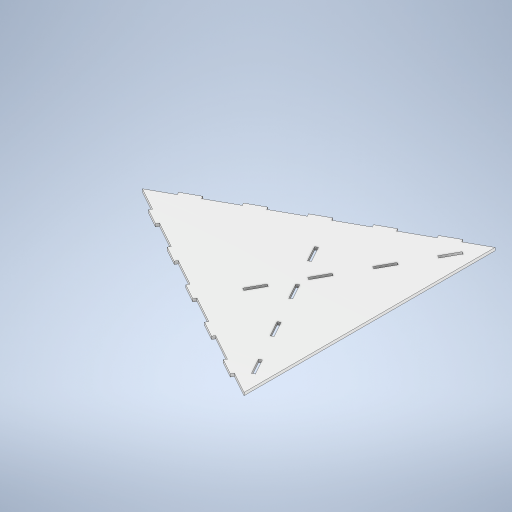
# Autodesk Inventor part: chair seat
Saved by Autodesk Inventor 2023 (Build 270158000, 158)
## iProperties
Created: 2023-09-18
Part Number: chair seat
Material: Polystyrene
Document SubType Name: Modeling
Designer: Nate
Density: 1.021 g/cm^3
Appearance: Smooth - White
Mass: 389.764 g
Surface Area: 1695.75 cm^2
Volume: 381.748 cm^3
Author: Nate
Autodesk Inventor part; units mm, degrees
ref_plane "YZ Plane" through (0, 0, 0) normal (1, 0, 0) x (0, 1, 0)
ref_plane "XZ Plane" through (0, 0, 0) normal (0, 1, 0) x (-1, 0, 0)
ref_plane "XY Plane" through (0, 0, 0) normal (0, 0, 1) x (1, 0, 0)
sketch "Sketch1" plane through (0, 0, 0) normal (0, 1, 0) x (-1, 0, 0)
  line L0 (-3.6958, 214.582) -> (-3.6958, -205.418)
  line L1 (-3.6958, 214.582) -> (376.3042, 4.582)
  line L2 (-3.6958, -205.418) -> (376.3042, 4.582)
  line L3 (-3.6958, 214.582) -> (174.1079, -107.158)
  line L4 (-3.6958, -205.418) -> (174.1079, 116.3221)
  line L5 (17.7358, 180.7241) -> (13.5674, 178.4206)
  line L6 (13.5674, 178.4206) -> (28.078, 152.1633)
  line L7 (28.078, 152.1633) -> (32.2464, 154.4669)
  line L8 (32.2464, 154.4669) -> (17.7358, 180.7241)
  line L9 (56.4307, 110.7048) -> (52.2623, 108.4013)
  line L10 (52.2623, 108.4013) -> (66.7729, 82.144)
  line L11 (66.7729, 82.144) -> (70.9413, 84.4476)
  line L12 (70.9413, 84.4476) -> (56.4307, 110.7048)
  line L13 (95.1256, 40.6855) -> (90.9572, 38.3819)
  line L14 (90.9572, 38.3819) -> (105.4678, 12.1247)
  line L15 (105.4678, 12.1247) -> (109.6361, 14.4282)
  line L16 (109.6361, 14.4282) -> (95.1256, 40.6855)
  line L17 (133.8205, -29.3338) -> (129.6521, -31.6374)
  line L18 (129.6521, -31.6374) -> (144.1627, -57.8946)
  line L19 (144.1627, -57.8946) -> (148.331, -55.5911)
  line L20 (148.331, -55.5911) -> (133.8205, -29.3338)
  line L21 (32.2464, -145.3028) -> (28.078, -142.9993)
  line L22 (28.078, -142.9993) -> (13.5674, -169.2565)
  line L23 (13.5674, -169.2565) -> (17.7358, -171.5601)
  line L24 (17.7358, -171.5601) -> (32.2464, -145.3028)
  line L25 (70.9413, -75.2835) -> (66.7729, -72.98)
  line L26 (66.7729, -72.98) -> (52.2623, -99.2372)
  line L27 (52.2623, -99.2372) -> (56.4307, -101.5408)
  line L28 (56.4307, -101.5408) -> (70.9413, -75.2835)
  line L29 (109.6361, -5.2642) -> (105.4678, -2.9606)
  line L30 (105.4678, -2.9606) -> (90.9572, -29.2179)
  line L31 (90.9572, -29.2179) -> (95.1256, -31.5214)
  line L32 (95.1256, -31.5214) -> (109.6361, -5.2642)
  line L33 (148.331, 64.7551) -> (144.1627, 67.0587)
  line L34 (144.1627, 67.0587) -> (129.6521, 40.8014)
  line L35 (129.6521, 40.8014) -> (133.8204, 38.4979)
  line L36 (133.8204, 38.4979) -> (148.331, 64.7551)
  point P0 (-3.6958, 4.582)
  point P1 (30.1622, 153.3151)
  point P2 (68.8571, 83.2958)
  point P3 (107.552, 13.2765)
  point P4 (146.2469, -56.7429)
  point P5 (30.1622, -144.1511)
  point P6 (146.2469, 65.9069)
  point P7 (107.552, -4.1124)
  point P8 (68.8571, -74.1317)
  dimension "d2" = 420
  dimension "d5" = 380
  dimension "d6" = 57.853
  dimension "d7" = 4.7625
  dimension "d8" = 30
  dimension "d9" = 4.7625
  dimension "d10" = 30
  dimension "d11" = 4.7625
  dimension "d12" = 30
  dimension "d13" = 4.7625
  dimension "d14" = 30
  dimension "d15" = 50
  dimension "d16" = 50
  dimension "d17" = 40
  dimension "d18" = 50
  dimension "d33" = 4.7625
  dimension "d35" = 30
  dimension "d36" = 4.7625
  dimension "d37" = 30
  dimension "d38" = 4.7625
  dimension "d39" = 30
  dimension "d40" = 4.7625
  dimension "d41" = 30
  dimension "d43" = 50
  dimension "d44" = 50
  dimension "d45" = 50
  dimension "d46" = 40
  constraints: 74 end point, 20 parallel, 10 perpendicular, 10 point on line, 9 midpoint, 1 vertical
  measures "d2" distance of L0.start L0.end
  measures "d5" distance of L1.end point (-3.696, 4.582)
  measures "d6" angle of L1 L2
  measures "d7" distance of L7.end L6.end
  measures "d8" distance of L6.end L5.end
  measures "d9" distance of L12.start L10.end
  measures "d10" distance of L10.end L9.end
  measures "d11" distance of L16.start L14.end
  measures "d12" distance of L14.end L13.end
  measures "d13" distance of L20.start L18.end
  measures "d14" distance of L18.end L17.end
  measures "d15" distance between parallel lines of L9 L7
  measures "d16" distance between parallel lines of L13 L11
  measures "d17" distance from line of L5 L0.start
  measures "d18" distance between parallel lines of L17 L15
  measures "d33" distance of L23.end L22.end
  measures "d35" distance between parallel lines of L23 L21
  measures "d36" distance of L28.start L26.end
  measures "d37" distance between parallel lines of L27 L25
  measures "d38" distance of L32.start L30.end
  measures "d39" distance between parallel lines of L31 L29
  measures "d40" distance of L36.start L34.end
  measures "d41" distance between parallel lines of L35 L33
  measures "d43" distance between parallel lines of L27 L21
  measures "d44" distance between parallel lines of L25 L31
  measures "d45" distance between parallel lines of L29 L35
  measures "d46" distance from line of L0.end L23
extrude "Extrusion1" add sketch "Sketch1" along normal blind 4.7625 contours L3 L5 L6 L7 L9 L10 L11 L13 L14 L15 L4 L29 L30 L31 L25 L26 L27 L21 L22 L23 L0 | L1 L4 L33 L34 L35 L3 L15 L16 L13 L11 L12 L9 L7 L8 L5 | L4 L23 L24 L21 L27 L28 L25 L31 L32 L29 L3 L17 L18 L19 L2 | L1 L2 L3 L19 L20 L17 L4 L35 L36 L33
sketch "Sketch2" plane through (-376.3042, 0, 4.582) normal (-0.4836861, 0, 0.8752415) x (0.8752415, 0, 0.4836861)
  line L0 (43, 0) -> (73, 0)
  line L1 (73, 0) -> (73, 4.7625)
  line L2 (73, 4.7625) -> (43, 4.7625)
  line L3 (43, 4.7625) -> (43, 0)
  line L4 (0, 0) -> (434.1659, 0) projected
  line L5 (0, 0) -> (0, 4.7625) projected
  line L6 (123, 0) -> (153, 0)
  line L7 (153, 0) -> (153, 4.7625)
  line L8 (153, 4.7625) -> (123, 4.7625)
  line L9 (123, 4.7625) -> (123, 0)
  line L10 (203, 0) -> (233, 0)
  line L11 (233, 0) -> (233, 4.7625)
  line L12 (233, 4.7625) -> (203, 4.7625)
  line L13 (203, 4.7625) -> (203, 0)
  line L14 (283, 0) -> (313, 0)
  line L15 (313, 0) -> (313, 4.7625)
  line L16 (313, 4.7625) -> (283, 4.7625)
  line L17 (283, 4.7625) -> (283, 0)
  line L18 (363, 0) -> (393, 0)
  line L19 (393, 0) -> (393, 4.7625)
  line L20 (393, 4.7625) -> (363, 4.7625)
  line L21 (363, 4.7625) -> (363, 0)
  point P0 (327.1408, 0)
  point P1 (363, 0)
  point P2 (393, 0)
  point P3 (283, 0)
  point P4 (313, 0)
  point P5 (203, 0)
  point P6 (233, 0)
  point P7 (123, 0)
  point P8 (153, 0)
  dimension "d49" = 30
  dimension "d50" = 4.7625
  dimension "d51" = 43
  dimension "d52" = 30
  dimension "d53" = 4.7625
  dimension "d54" = 30
  dimension "d55" = 4.7625
  dimension "d56" = 30
  dimension "d57" = 4.7625
  dimension "d58" = 30
  dimension "d59" = 4.7625
  dimension "d60" = 50
  dimension "d61" = 50
  dimension "d62" = 50
  dimension "d63" = 50
  constraints: 40 end point, 10 parallel, 5 horizontal, 5 perpendicular, 1 collinear
  measures "d49" distance of L2.end L1.end
  measures "d50" distance of L1.end L0.end
  measures "d51" distance between parallel lines of L3 L5
  measures "d52" distance of L8.end L8.start
  measures "d53" distance of L8.start L6.end
  measures "d54" distance of L12.end L12.start
  measures "d55" distance of L12.start L10.end
  measures "d56" distance of L16.end L16.start
  measures "d57" distance of L16.start L14.end
  measures "d58" distance of L20.end L20.start
  measures "d59" distance of L20.start L18.end
  measures "d60" distance between parallel lines of L9 L1
  measures "d61" distance between parallel lines of L13 L7
  measures "d62" distance between parallel lines of L17 L11
  measures "d63" distance between parallel lines of L21 L15
extrude "Extrusion2" add sketch "Sketch2" along normal blind 5
sketch "Sketch3" plane through (3.6958, 0, -205.418) normal (-0.4836861, 0, -0.8752415) x (-0.8752415, 0, 0.4836861)
  line L0 (361.1659, 4.7625) -> (391.1659, 4.7625)
  line L1 (391.1659, 4.7625) -> (391.1659, 0)
  line L2 (391.1659, 0) -> (361.1659, 0)
  line L3 (361.1659, 0) -> (361.1659, 4.7625)
  line L4 (0, 0) -> (434.1659, 0) projected
  line L5 (281.1659, 4.7625) -> (311.1659, 4.7625)
  line L6 (311.1659, 4.7625) -> (311.1659, 0)
  line L7 (311.1659, 0) -> (281.1659, 0)
  line L8 (281.1659, 0) -> (281.1659, 4.7625)
  line L9 (201.1659, 4.7625) -> (231.1659, 4.7625)
  line L10 (231.1659, 4.7625) -> (231.1659, 0)
  line L11 (231.1659, 0) -> (201.1659, 0)
  line L12 (201.1659, 0) -> (201.1659, 4.7625)
  line L13 (121.1659, 4.7625) -> (151.1659, 4.7625)
  line L14 (151.1659, 4.7625) -> (151.1659, 0)
  line L15 (151.1659, 0) -> (121.1659, 0)
  line L16 (121.1659, 0) -> (121.1659, 4.7625)
  line L17 (41.1659, 4.7625) -> (71.1659, 4.7625)
  line L18 (71.1659, 4.7625) -> (71.1659, 0)
  line L19 (71.1659, 0) -> (41.1659, 0)
  line L20 (41.1659, 0) -> (41.1659, 4.7625)
  line L21 (434.1659, 0) -> (434.1659, 4.7625) projected
  point P0 (102.5926, 0)
  point P1 (281.1659, 0)
  point P2 (311.1659, 0)
  point P3 (201.1659, 0)
  point P4 (231.1659, 0)
  point P5 (121.1659, 0)
  point P6 (151.1659, 0)
  point P7 (41.1659, 0)
  point P8 (71.1659, 0)
  dimension "d66" = 30
  dimension "d67" = 4.7625
  dimension "d68" = 30
  dimension "d69" = 4.7625
  dimension "d70" = 30
  dimension "d71" = 4.7625
  dimension "d72" = 30
  dimension "d73" = 4.7625
  dimension "d74" = 30
  dimension "d75" = 4.7625
  dimension "d76" = 43
  dimension "d77" = 50
  dimension "d78" = 50
  dimension "d79" = 50
  dimension "d80" = 50
  constraints: 40 end point, 10 parallel, 5 horizontal, 5 perpendicular, 1 collinear
  measures "d66" distance of L1.end L2.end
  measures "d67" distance of L0.end L1.end
  measures "d68" distance of L6.end L8.start
  measures "d69" distance of L6.start L6.end
  measures "d70" distance of L10.end L12.start
  measures "d71" distance of L10.start L10.end
  measures "d72" distance of L14.end L16.start
  measures "d73" distance of L14.start L14.end
  measures "d74" distance of L18.end L20.start
  measures "d75" distance of L18.start L18.end
  measures "d76" distance between parallel lines of L21 L1
  measures "d77" distance between parallel lines of L3 L6
  measures "d78" distance between parallel lines of L8 L10
  measures "d79" distance between parallel lines of L12 L14
  measures "d80" distance between parallel lines of L16 L18
extrude "Extrusion3" add sketch "Sketch3" along normal blind 5
body "Solid1"
